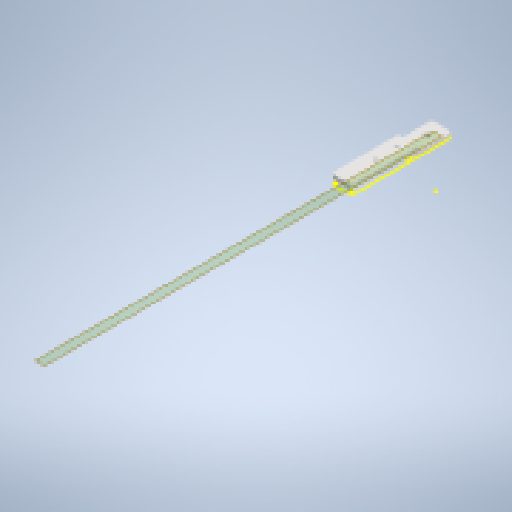
# Autodesk Inventor part: крепление шкива боковое
Saved by Autodesk Inventor 2024.2 (Build 282272000, 272)
## iProperties
Created: 2026-02-02
Part Number: крепление шкива боковое
Material: Типовые
Document SubType Name: Modeling
Designer: katya_notebook
Density: 1 g/cm^3
Appearance: По умолчанию
Author: katya_notebook
Autodesk Inventor part; units mm, degrees
ref_plane "YZ Plane" through (0, 0, 0) normal (1, 0, 0) x (0, 1, 0)
ref_plane "XZ Plane" through (0, 0, 0) normal (0, 1, 0) x (-1, 0, 0)
ref_plane "XY Plane" through (0, 0, 0) normal (0, 0, 1) x (1, 0, 0)
ref_plane "РабПлоскость1" through (-30.8415, -18.9359, 233.6055) normal (0, -1, 0) x (1, 0, 0)
sketch "Эскиз1" plane through (-30.8415, -18.9359, 233.6055) normal (0, -1, 0) x (1, 0, 0)
  line L0 (-13.3, -2.4998) -> (-13.3, -252.4998) projected
  line L1 (6.7, -2.4998) -> (6.7, -252.4998) projected
  line L2 (-13.3, -201.9768) -> (6.7, -201.9768)
  line L3 (6.7, -201.9768) -> (6.7, -265.9768)
  line L4 (0.7, -271.9768) -> (-7.3, -271.9768)
  line L5 (-13.3, -265.9768) -> (-13.3, -201.9768)
  line L6 (-6.6, -2.4998) -> (-6.6, -252.4998) projected
  line L7 (0, -2.4998) -> (0, -252.4998) projected
  circle A0 centre (-3.3, -240.4998) radius 1.25
  circle A1 centre (-3.3, -225.4998) radius 1.25
  line L8 (-6.2394, -252.4998) -> (-3.6, -252.4998) projected
  arc A2 (-13.3, -265.9768) -> (-7.3, -271.9768) centre (-7.3, -265.9768) ccw
  arc A3 (0.7, -271.9768) -> (6.7, -265.9768) centre (0.7, -265.9768) ccw
  circle A4 centre (-3.3, -260.4999) radius 3.3 projected
  point P0 (30.8415, -233.6055)
  point P1 (-13.3, -271.9768)
  point P2 (-4.9197, -252.4998)
  dimension "d0" = 70
  dimension "d1" = 15
  dimension "d2" = 2.5
  dimension "d3" = 2.5
  dimension "d4" = 3.3
  dimension "d5" = 12
  dimension "d6" = 6
  constraints: 8 end point, 4 centre point, 4 point on circle, 4 point on line, 4 tangent, 2 parallel, 1 equal radius, 1 horizontal, 1 midpoint, 1 perpendicular, 1 vertical alignment
  measures "d0" distance of point (-13.3, -271.977) L2.start
  measures "d1" distance of A1.centre A0.centre
  measures "d2" diameter of A0
  measures "d3" diameter of A1
  measures "d4" distance from line of L6 A1.centre
  measures "d5" vertical distance of point (-4.92, -252.5) A0.centre
  measures "d6" radius of A2
extrude "Выдавливание1" add sketch "Эскиз1" along normal blind 3
sketch "Эскиз2" plane through (-30.8415, -21.9359, 233.6055) normal (0, -1, 0) x (1, 0, 0)
  line L0 (-13.3, -201.9768) -> (-13.3, -265.9768) projected
  line L1 (-13.3, -248.5067) -> (-13.3, -271.9768)
  line L2 (-13.3, -271.9768) -> (6.7, -271.9768)
  line L3 (6.7, -271.9768) -> (6.7, -248.5067)
  line L4 (6.7, -265.9768) -> (6.7, -201.9768) projected
  line L5 (-13.3, -248.5067) -> (6.7, -248.5067)
  point P0 (30.8415, -233.6055)
  point P1 (0.7, -271.9768)
  constraints: 8 end point, 3 point on line, 2 perpendicular, 2 vertical, 1 collinear, 1 horizontal
extrude "Выдавливание2" cut sketch "Эскиз2" against normal blind 3
sketch "Эскиз3" plane through (-30.8415, -21.9359, 233.6055) normal (0, -1, 0) x (1, 0, 0)
  line L0 (-13.3, -201.9768) -> (-13.3, -248.5067) projected
  line L1 (-13.3, -244.5067) -> (6.7, -244.5067)
  line L2 (6.7, -244.5067) -> (6.7, -271.5067)
  line L3 (6.7, -271.5067) -> (-13.3, -271.5067)
  line L4 (-13.3, -271.5067) -> (-13.3, -244.5067)
  line L5 (6.7, -248.5067) -> (6.7, -201.9768) projected
  line L6 (-13.3, -248.5067) -> (6.7, -248.5067) projected
  circle A0 centre (-3.3, -260.4998) radius 2.5 projected
  circle A1 centre (-3.3, -260.4998) radius 2.25
  point P0 (30.8415, -233.6055)
  dimension "d11" = 27
  dimension "d12" = 4
  dimension "d22" = 4.5
  constraints: 8 end point, 2 parallel, 2 point on line, 1 centre point, 1 coincident, 1 horizontal, 1 perpendicular
  measures "d11" distance of L3.end L1.start
  measures "d12" distance between parallel lines of L6 L1
  measures "d22" diameter of A1
extrude "Выдавливание3" add sketch "Эскиз3" along normal blind 3 contours L1 L2 L6 L0 | L6 L2 L3 L4 | A0
fillet "Сопряжение1" radius 3 3 edges at (-34.1415, -21.9359, -10.9012) (-34.1415, -21.9359, -14.9012) (-34.1415, -24.9359, -10.9012)
fillet "Сопряжение2" radius 3 4 edges at (-44.1415, -23.4359, -37.9012) (-24.1415, -23.4359, -37.9012) (-44.1415, -20.4359, 31.6287) (-24.1415, -20.4359, 31.6287)
sketch "Эскиз4" plane through (-30.8415, -21.9359, 233.6055) normal (0, -1, 0) x (1, 0, 0)
  arc A0 (3.7, -271.5067) -> (6.7, -268.5067) centre (3.7, -268.5067) ccw projected
  line L0 (3.7, -271.5067) -> (6.7, -271.5067)
  line L1 (6.7, -271.5067) -> (6.7, -201.9768)
  line L2 (6.7, -201.9768) -> (3.7, -201.9768)
  line L3 (3.7, -201.9768) -> (3.7, -271.5067)
  arc A1 (-13.3, -268.5067) -> (-10.3, -271.5067) centre (-10.3, -268.5067) ccw projected
  line L4 (-10.3, -271.5067) -> (-13.3, -271.5067)
  line L5 (-13.3, -271.5067) -> (-13.3, -201.9768)
  line L6 (-13.3, -201.9768) -> (-10.3, -201.9768)
  line L7 (-10.3, -201.9768) -> (-10.3, -271.5067)
  point P0 (30.8415, -233.6055)
  point P1 (-13.3, -268.5067)
  point P2 (6.7, -268.5067)
  constraints: 16 end point, 4 parallel, 2 horizontal, 2 perpendicular, 1 point on line
extrude "Выдавливание4" cut sketch "Эскиз4" along normal blind 10 and the other way blind 5 contours L3 L2 L1 A0 | L5 L6 L7 A1
fillet "Сопряжение3" radius 2 4 edges at (-41.1415, -23.4359, -37.9012) (-27.1415, -23.4359, -37.9012) (-27.1415, -20.4359, 31.6287) (-41.1415, -20.4359, 31.6287)
sketch "Эскиз5" plane through (-30.8415, -24.9359, 233.6055) normal (0, -1, 0) x (1, 0, 0)
  arc A0 (1.7, -271.5067) -> (3.7, -269.5067) centre (1.7, -269.5067) ccw projected
  line L0 (3.7, -269.5067) -> (3.7, -247.5067) projected
  line L1 (-10.3, -247.5067) -> (3.7, -247.5067) projected
  line L2 (-10.3, -247.5067) -> (-10.3, -269.5067) projected
  arc A1 (-10.3, -269.5067) -> (-8.3, -271.5067) centre (-8.3, -269.5067) ccw projected
  line L3 (-8.3, -271.5067) -> (1.7, -271.5067) projected
  circle A2 centre (-3.3, -260.4998) radius 2.25 projected
  arc A3 (-8.3, -201.9768) -> (-10.3, -203.9768) centre (-8.3, -203.9768) ccw projected
  line L4 (-10.3, -203.9768) -> (-10.3, -242.3106) projected
  line L5 (3.7, -242.3106) -> (-10.3, -242.3106) projected
  line L6 (3.7, -242.3106) -> (3.7, -203.9768) projected
  arc A4 (3.7, -203.9768) -> (1.7, -201.9768) centre (1.7, -203.9768) ccw projected
  line L7 (1.7, -201.9768) -> (-8.3, -201.9768) projected
  circle A5 centre (-3.3, -225.4998) radius 1.25 projected
  circle A6 centre (-3.3, -240.4998) radius 1.25 projected
  line L8 (-10.3, -242.3106) -> (-10.3, -244.9086) projected
  line L9 (-10.3, -244.9086) -> (3.7, -244.9086) projected
  line L10 (3.7, -244.9086) -> (3.7, -242.3106) projected
  line L11 (3.7, -242.3106) -> (-10.3, -242.3106) projected
  line L12 (-10.3, -244.9086) -> (-10.3, -247.5067) projected
  line L13 (-10.3, -247.5067) -> (3.7, -247.5067) projected
  line L14 (3.7, -247.5067) -> (3.7, -244.9086) projected
  line L15 (-10.3, -244.9086) -> (3.7, -244.9086) projected
  point P0 (30.8415, -233.6055)
